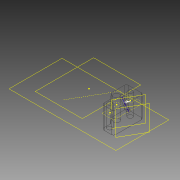
# Autodesk Inventor part: CLOSESTOPBRKT
Saved by Autodesk Inventor 2015 (Build 190159000, 159)
## iProperties
Created: 2015-09-18
Part Number: CLOSESTOPBRKT
Material: Generic
Description: insert part description/title
Document SubType Name: Modeling
Designer: francis
Density: 1 g/cm^3
Appearance: Default
Part Category: insert part category here and press enter to fill value
Author: francis
Autodesk Inventor part; units mm, degrees
ref_plane "YZ Plane" through (0, 0, 0) normal (1, 0, 0) x (0, 1, 0)
ref_plane "XZ Plane" through (0, 0, 0) normal (0, 1, 0) x (-1, 0, 0)
ref_plane "XY Plane" through (0, 0, 0) normal (0, 0, 1) x (1, 0, 0)
ref_plane "Work Plane1" through (0, 0, 0) normal (0, 0, 1) x (1, 0, 0)
ref_plane "Work Plane2" through (-37, -13, 19) normal (0, 0, -1) x (0, 1, 0)
sketch "Sketch1" plane through (0, 0, 0) normal (0, 0, 1) x (1, 0, 0)
  line L0 (35, 13.1624) -> (35, -13.1624) projected
  line L1 (20, -13.1624) -> (20, 13.1624) projected
  circle A0 centre (27.5, 9) radius 2 projected
  circle A1 centre (27.5, -9) radius 2 projected
  circle A2 centre (24.5, 0) radius 2.5
  line L2 (35, 13.1624) -> (20, 13.1624)
  line L3 (35, -13.1624) -> (24.5, -13.1624)
  line L4 (24.5, -13.1624) -> (24.5, -5.5685)
  line L5 (24.5, -5.5685) -> (20, 0)
  line L6 (20, 0) -> (20, 13.1624)
  point P0 (0, 0)
  dimension "d0" = 3.5
  dimension "d1" = 3
  dimension "d25" = 5
  constraints: 10 end point, 2 horizontal, 1 centre point, 1 collinear, 1 midpoint, 1 perpendicular
  measures "d0" distance from line of L5 A2.centre
  measures "d1" distance from line of L4 A1.centre
  measures "d25" diameter of A2
extrude "Extrusion1" add sketch "Sketch1" along normal up to surface (19 mm away)
ref_plane "Work Plane4" through (-0.8627, 0, 12) normal (0, 0, 1) x (1, 0, 0)
sketch "Sketch4" plane through (-0.8627, 0, 12) normal (0, 0, 1) x (1, 0, 0)
  circle A0 centre (28.3627, 9) radius 2 construction
  circle A1 centre (25.3627, 0) radius 2.5 construction
  circle A2 centre (28.3627, -9) radius 2 construction
  circle A3 centre (25.3627, 0) radius 2.5 construction
  circle A4 centre (28.3627, -9) radius 2 construction
  circle A5 centre (28.3627, 9) radius 2 construction
  line L0 (35.8627, -13.1624) -> (35.8627, 13.1624) construction
  line L1 (35.8627, 13.1624) -> (20.8627, 13.1624) construction
  line L2 (20.8627, 13.1624) -> (20.8627, 0) construction
  line L3 (20.8627, 0) -> (25.3627, -5.5685) construction
  line L4 (25.3627, -5.5685) -> (25.3627, -13.1624) construction
  line L5 (25.3627, -13.1624) -> (35.8627, -13.1624) construction
  line L6 (20.8627, 8.7113) -> (35.8627, 0.0511) construction
  line L7 (35.8627, -13.1624) -> (35.8627, 13.1624) construction
  line L8 (-2.1421, -20.2045) -> (16.8579, 12.7045) construction
  line L9 (35.8627, 0.0511) -> (20.8627, 8.7113)
  point P0 (0.8627, 0)
  dimension "d6" = 4
  constraints: 4 end point, 2 point on line, 1 perpendicular
  measures "d6" distance from line of A0.centre L6
ref_plane "Work Plane8" through (43.6603, -4.9489, 12) normal (0.8660254, -0.5, 0) x (0.5, 0.8660254, 0)
ref_plane "Work Plane7" through (35, 0.0511, 12) normal (0.8660254, -0.5, 0) x (0.5, 0.8660254, 0)
sketch "Sketch7" plane through (43.6603, -4.9489, 12) normal (0.8660254, -0.5, 0) x (0.5, 0.8660254, 0)
  point P0 (-17.5442, -12)
  point P1 (0, 0)
hole "Hole2" at (43.6603, -4.9489, 12) direction (-0.8660254, 0.5, 0) diameter 2.459 end through all thread size "M3x0.5" class "6H" standard "ISO Metric profile"
fillet "Fillet1" radius 2 4 edges at (35, 13.1624, 9.5) (20, 13.1624, 9.5) (24.5, -13.1624, 9.5) (35, -13.1624, 9.5)
body "Solid1"
